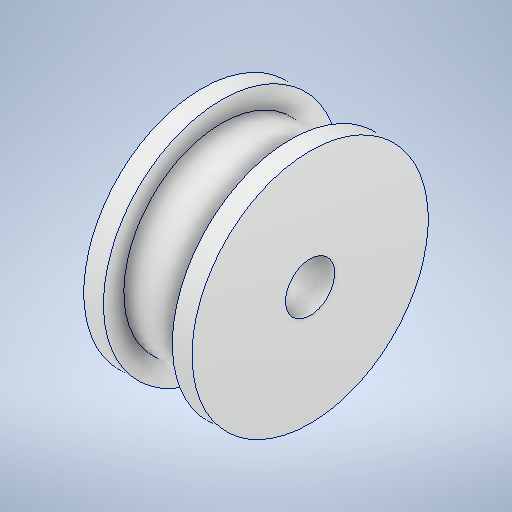
# Autodesk Inventor part: Belt_Pulley
Saved by Autodesk Inventor 2025.1 (Build 291241020, 241B)
## iProperties
Created: 2024-11-07
Part Number: Belt_Pulley
Material: Aluminum 6061
Document SubType Name: Modeling
Designer: leon-
Density: 2.7 g/cm^3
Appearance: Aluminum - Flat
Author: leon-
Autodesk Inventor part; units mm, degrees
ref_plane "YZ Plane" through (0, 0, 0) normal (1, 0, 0) x (0, 1, 0)
ref_plane "XZ Plane" through (0, 0, 0) normal (0, 1, 0) x (-1, 0, 0)
ref_plane "XY Plane" through (0, 0, 0) normal (0, 0, 1) x (1, 0, 0)
sketch "Sketch1" plane through (0, 0, 0) normal (0, 0, 1) x (1, 0, 0)
  line L0 (5.5, 2.5) -> (5.5, 12)
  line L1 (5.5, 12) -> (3.5, 12)
  line L2 (3.5, 12) -> (3.5, 9.93)
  line L3 (3.5, 9.93) -> (0, 9.93)
  line L4 (5.5, 2.5) -> (0, 2.5)
  line L5 (0, 2.5) -> (0, 9.93)
  line L6 (-2.3, 0) -> (6.8, 0) projected
  line L7 (0, 0) -> (0, 17.5) projected
  line L8 (0, 9) -> (0, 2.5)
  line L9 (0, 15) -> (0, 9)
  point P0 (0, 6.215)
  point P1 (-1, 12)
  point P2 (4.5, 12)
  dimension "d0" = 5.5
  dimension "d1" = 3.5
  dimension "d2" = 9.93
  dimension "d3" = 12
  dimension "d4" = 2.5
  dimension "d8" = 1
  constraints: 16 end point, 4 perpendicular, 2 midpoint, 1 collinear, 1 horizontal, 1 vertical
  measures "d0" distance between parallel lines of L5 L0
  measures "d1" distance from line of point (0, 6.215) L2
  measures "d2" distance between parallel lines of L6 L3
  measures "d3" distance between parallel lines of L6 L1
  measures "d4" distance between parallel lines of L6 L4
  measures "d8" distance from line of L5 point (-1, 12)
revolve "Revolution1" add sketch "Sketch1" angle 360 about axis through (-10, 0, 0) along (1, 0, 0)
mirror "Mirror2" about plane through (0, 0, 0) normal (1, 0, 0) of "Revolution1"
body "Solid1"
